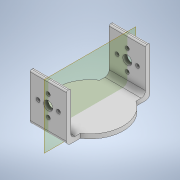
# Autodesk Inventor part: мотор_локтя_2
Saved by Autodesk Inventor 2022 (Build 260153000, 153)
## iProperties
Created: 2022-12-04
Part Number: мотор_локтя_2
Material: Типовые
Document SubType Name: Modeling
Designer: Папа
Density: 1 g/cm^3
Appearance: По умолчанию
Author: Папа
Autodesk Inventor part; units mm, degrees
ref_plane "YZ Plane" through (0, 0, 0) normal (1, 0, 0) x (0, 1, 0)
ref_plane "XZ Plane" through (0, 0, 0) normal (0, 1, 0) x (-1, 0, 0)
ref_plane "XY Plane" through (0, 0, 0) normal (0, 0, 1) x (1, 0, 0)
sketch "Эскиз1" plane through (0, 0, 0) normal (0, 1, 0) x (-1, 0, 0)
  line L0 (-12.5, 25.75) -> (12.5, 25.75)
  line L1 (12.5, 25.75) -> (12.5, -25.75)
  line L2 (12.5, -25.75) -> (-12.5, -25.75)
  line L3 (-12.5, -25.75) -> (-12.5, 25.75)
  line L4 (-12.5, 25.75) -> (12.5, -25.75) construction
  line L5 (12.5, 25.75) -> (-12.5, -25.75) construction
  circle A0 centre (0, 0) radius 22.9
  point P0 (-12.5, 19.1875)
  point P1 (-12.5, -19.1875)
  point P2 (12.5, -19.1875)
  point P3 (12.5, 19.1875)
  dimension "d0" = 51.5
  dimension "d1" = 25
  dimension "d2" = 45.8
  constraints: 12 end point, 2 midpoint, 2 parallel, 1 centre point, 1 coincident, 1 horizontal, 1 perpendicular
  measures "d0" distance of L0.end L1.end
  measures "d1" distance of L1.end L2.end
  measures "d2" diameter of A0
extrude "Выдавливание1" add sketch "Эскиз1" along normal blind 3
sketch "Эскиз2" plane through (0, 0, 0) normal (0, -1, 0) x (1, 0, 0)
  circle A0 centre (0, 0) radius 20.9
  circle A1 centre (0, 0) radius 18.9
  dimension "d6" = 37.8
  dimension "d7" = 2
  constraints: 2 centre point, 2 coincident
  measures "d6" diameter of A1
  measures "d7" radial gap between concentric circles of A0 A1
extrude "Выдавливание2" add sketch "Эскиз2" along normal blind 1
fillet "Сопряжение1" radius 2 1 edges at (-20.9, 0, 0)
sketch "Эскиз3" plane through (0, 0, 0) normal (0, -1, 0) x (1, 0, 0)
  circle A0 centre (0, 0) radius 12.35
  dimension "d13" = 24.7
  constraints: 1 centre point, 1 coincident
  measures "d13" diameter of A0
extrude "Выдавливание3" add sketch "Эскиз3" along normal blind 7
sketch "Эскиз4" plane through (0, -7, 0) normal (0, -1, 0) x (1, 0, 0)
  circle A0 centre (0, 0) radius 12.35 projected
  circle A1 centre (0, 0) radius 12.6
  line L0 (0, 0) -> (0.3298, -12.5957)
  line L1 (0, 0) -> (-0.3298, -12.5957)
  line L2 (0.3298, -12.5957) -> (-0.3298, -12.5957) construction
  point P0 (-0.3233, -12.3458)
  point P1 (0.3233, -12.3458)
  dimension "d44" = 3
  dimension "d45" = 0.25
  constraints: 6 end point, 2 point on circle, 1 centre point, 1 coincident, 1 horizontal
  measures "d44" angle of L1 L0
  measures "d45" radial gap between concentric circles of A0 A1
extrude "Выдавливание4" add sketch "Эскиз4" against normal up to surface (7 mm away) contours A0 L0 A1 L1 picked at (-0.2543, -12.5137)
fillet "Сопряжение4" radius 0.7 2 edges at (-0.3233, -3.5, -12.3458) (0.3233, -3.5, -12.3458)
fillet "Сопряжение10" radius 0.3 2 edges at (0.3298, -3.5, -12.5957) (-0.3298, -3.5, -12.5957)
pattern_circular "Круговой массив1" count 8 over 360 about axis through (0, 0, 0) along (0, -1, 0) of "Выдавливание4", "Сопряжение4"
fillet "Сопряжение5" radius 0.2 19 edges at (-11.4099, -7, -4.7261) (-4.7261, -7, -11.4099) (-11.4099, -7, 4.7261) (-4.7261, -7, 11.4099) (4.7261, -7, 11.4099) (11.4099, -7, 4.7261) (11.4099, -7, -4.7261) (4.7261, -7, -11.4099) (-11.4099, 0, -4.7261) (-11.4099, 0, 4.7261) (-4.7261, 0, 11.4099) (4.7261, 0, 11.4099) (11.4099, 0, 4.7261) (11.4099, 0, -4.7261) (4.7261, 0, -11.4099) (-4.7261, 0, -11.4099) (-18.9, 0, 0) (-18.9, -1, 0) (-20.9, -1, 0)
ref_plane "РабПлоскость1" through (-12.5, 0, 0) normal (0, 0, 1) x (1, 0, 0)
sketch "Эскиз6" plane through (-12.5, 0, 25.75) normal (0, 0, 1) x (1, 0, 0)
  line L0 (0, 0) -> (25, 0)
  line L1 (25, 0) -> (25, 3)
  line L2 (25, 3) -> (0, 3)
  line L3 (0, 3) -> (0, 0)
  line L4 (0, 3) -> (25, 3) projected
  line L5 (0, 0) -> (0, 3) projected
  line L6 (0, 3) -> (25, 3)
  line L7 (25, 3) -> (25, 33)
  line L8 (25, 33) -> (0, 33)
  line L9 (0, 33) -> (0, 3)
  line L10 (25, 3) -> (0, 3) projected
  line L11 (0, 33) -> (25, 3) construction
  circle A0 centre (12.5, 18) radius 3.1
  line L12 (25, 0) -> (25, 3) projected
  point P0 (12.5, 0)
  point P1 (25, 3)
  point P2 (25, 3)
  dimension "d25" = 30
  dimension "d26" = 6.2
  constraints: 18 end point, 4 parallel, 3 collinear, 2 horizontal, 2 perpendicular, 1 centre point, 1 midpoint
  measures "d25" distance between parallel lines of L2 L8
  measures "d26" diameter of A0
extrude "Выдавливание5" add sketch "Эскиз6" along normal blind 3
fillet "Сопряжение6" radius 3 1 edges at (0, 3, 25.75)
fillet "Сопряжение7" radius 1 2 edges at (0, 33, 28.75) (0, 33, 25.75)
mirror "Зеркальное отражение1" about plane through (-12.5, 0, 0) normal (0, 0, 1) of "Выдавливание5", "Сопряжение7", "Сопряжение6"
fillet "Сопряжение8" radius 3 2 edges at (0, 0, 28.75) (0, 0, -28.75)
sketch "Эскиз7" plane through (12.5, 32, -28.75) normal (0, 0, -1) x (-1, 0, 0)
  circle A0 centre (12.5, -14) radius 3.1 construction
  circle A1 centre (12.5, -14) radius 3.1 construction
  circle A2 centre (19.5, -14) radius 1.35
  line L0 (19.5, -14) -> (12.5, -14) construction
  circle A3 centre (12.5, -7) radius 1.35
  circle A4 centre (5.5, -14) radius 1.35
  circle A5 centre (12.5, -21) radius 1.35
  point P0 (12.5, -32)
  dimension "d32" = 2.7
  dimension "d33" = 7
  dimension "d36" = 360
  constraints: 5 centre point, 2 end point, 1 coincident, 1 horizontal, 9 other
  measures "d32" diameter of A2
  measures "d33" distance of L0.start L0.end
extrude "Выдавливание6" cut sketch "Эскиз7" against normal blind 3000
sketch "Эскиз8" plane through (0, -7, 0) normal (0, -1, 0) x (1, 0, 0)
  arc A0 (9.3116, -8.414) -> (12.5339, -0.6347) centre (0, 0) ccw projected
  circle A1 centre (0, 0) radius 2.5
  dimension "d40" = 5
  constraints: 1 centre point, 1 coincident
  measures "d40" diameter of A1
extrude "Выдавливание7" cut sketch "Эскиз8" against normal blind 2
fillet "Сопряжение9" radius 0.3 2 edges at (-2.5, -5, 0) (-2.5, -7, 0)
ref_plane "РабПлоскость2" through (0, 0, -19.1875) normal (-1, 0, 0) x (0, 0, 1)
sketch "Эскиз9" plane through (0, 0, -19.1875) normal (-1, 0, 0) x (0, 0, 1)
  line L0 (19.0967, -7) -> (18.362, -7) projected
  line L1 (19.0967, -7) -> (19.2783, -7) projected
  line L2 (20.013, -7) -> (19.2783, -7) projected
  line L3 (27.1753, -7) -> (20.013, -7) projected
  line L4 (28.0326, -7) -> (27.1753, -7) projected
  line L5 (28.0326, -7) -> (28.161, -7) projected
  line L6 (28.3427, -7) -> (28.161, -7) projected
  line L7 (31.3094, -7) -> (28.3427, -7) projected
  line L8 (31.7872, -7) -> (31.3094, -7) projected
  line L9 (31.7872, -7) -> (31.7872, -7) projected
  line L10 (31.3094, -7) -> (31.7872, -7) projected
  line L11 (28.3427, -7) -> (31.3094, -7) projected
  line L12 (28.161, -7) -> (28.3427, -7) projected
  line L13 (28.161, -7) -> (28.0326, -7) projected
  line L14 (27.1753, -7) -> (28.0326, -7) projected
  line L15 (20.013, -7) -> (27.1753, -7) projected
  line L16 (19.2783, -7) -> (20.013, -7) projected
  line L17 (19.2783, -7) -> (19.0967, -7) projected
  line L18 (18.362, -7) -> (19.0967, -7) projected
  line L19 (11.1997, -7) -> (18.362, -7) projected
  line L20 (10.3424, -7) -> (11.1997, -7) projected
  line L21 (10.3424, -7) -> (10.214, -7) projected
  line L22 (10.0323, -7) -> (10.214, -7) projected
  line L23 (7.0656, -7) -> (10.0323, -7) projected
  line L24 (6.8169, -7) -> (7.0656, -7) projected
  line L25 (6.789, -7) -> (6.8169, -7) projected
  line L26 (6.789, -7) -> (6.789, -7) projected
  line L27 (6.8169, -7) -> (6.789, -7) projected
  line L28 (7.0656, -7) -> (6.8169, -7) projected
  line L29 (10.0323, -7) -> (7.0656, -7) projected
  line L30 (10.214, -7) -> (10.0323, -7) projected
  line L31 (10.214, -7) -> (10.3424, -7) projected
  line L32 (11.1997, -7) -> (10.3424, -7) projected
  line L33 (18.362, -7) -> (11.1997, -7) projected
  line L34 (16.3875, -7) -> (21.9875, -7) projected
  line L35 (6.5875, -6.8) -> (6.5875, -0.2) projected
  line L36 (6.5875, -7) -> (7.1875, -7)
  line L37 (7.1875, -7) -> (7.1875, -6.4) construction
  line L38 (7.1875, -6.4) -> (6.5875, -6.4) construction
  line L39 (6.5875, -6.4) -> (6.5875, -7)
  line L40 (7.1875, -7) -> (6.5875, -6.4)
  line L41 (19.1875, -15) -> (19.1875, 41) projected
  point P0 (19.1875, 0)
  point P1 (7.1875, -7)
  point P2 (6.5875, -6.4)
  point P3 (6.5875, -6.8)
  point P4 (6.789, -7)
  dimension "d49" = 0.6
  constraints: 10 end point, 2 collinear, 2 parallel, 2 perpendicular, 1 horizontal
  measures "d49" distance of L37.end L38.end
revolve "Вращение1" cut sketch "Эскиз9" angle 360 about axis through (0, -10, 0) along (0, 1, 0)
